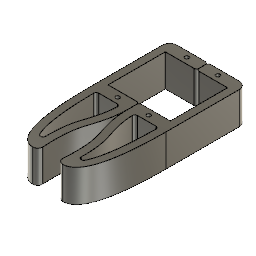
leg2 (Autodesk Fusion 360 design; units mm, degrees)
Autodesk Fusion 360 part; units mm, degrees
sketch "Sketch1" plane through (0, 0, 0) normal (0, 0, 1) x (1, 0, 0)
  line L0 (5.25, 11.5) -> (-6.25, 11.5)
  line L1 (-6.25, 11.5) -> (-6.25, -11.5)
  line L2 (-6.25, -11.5) -> (5.25, -11.5)
  line L3 (-9.25, 13.25) -> (-9.25, -16.25)
  line L4 (6.25, 12.5) -> (6.25, 15.25)
  line L5 (6.25, -12.5) -> (6.25, -16.25)
  line L6 (5.25, 16.25) -> (-6.25, 16.25)
  circle A0 centre (0, 13.9) radius 0.8
  circle A1 centre (0, -13.9) radius 0.8
  spline S0 degree 5 poles (6.25, -16.25) (6.25, -16.6676) (6.2357, -17.5036) (6.1715, -18.7605) (6.0031, -20.434) (5.6739, -22.4784) (5.2523, -24.4268) (4.7694, -26.2419) (4.2577, -27.9159) (3.7493, -29.4897) (3.2734, -31.0346) (2.8556, -32.634) (2.516, -34.367) (2.2668, -36.2872) (2.1131, -38.4227) (2.0561, -40.7853) (2.087, -42.8585) (2.1522, -44.515) (2.2143, -45.6642) (2.25, -46.25) knots 0 0 0 0 0 0 0.066667 0.133333 0.2 0.266667 0.333333 0.4 0.466667 0.533333 0.6 0.666667 0.733333 0.8 0.866667 0.933333 1 1 1 1 1 1
  arc A2 (0.25, -48.25) -> (2.25, -46.25) centre (0.25, -46.25) ccw
  spline S1 degree 5 poles (-9.25, -16.25) (-9.25, -17.2508) (-9.2353, -19.2506) (-9.1693, -22.2447) (-8.9897, -26.2076) (-8.5912, -31.003) (-7.9895, -35.4883) (-7.1545, -39.4912) (-6.0655, -42.8464) (-4.722, -45.4219) (-3.1673, -47.1742) (-1.8215, -47.9565) (-0.7899, -48.2233) (-0.0974, -48.264) (0.25, -48.25) knots 0 0 0 0 0 0 0.1 0.2 0.3 0.4 0.5 0.6 0.7 0.8 0.9 1 1 1 1 1 1
  line L7 (6.25, -13) -> (6.25, -19.5)
  line L8 (-9.25, -12) -> (-9.25, -20.5)
  line L9 (-2.6364, -48.3662) -> (3.1364, -48.1338)
  spline S2 degree 3 poles (-6.2471, -17.2558) (-6.2233, -21.3469) (-6.0529, -25.437) (-5.6953, -29.2432) (-5.3067, -33.3791) (-4.6726, -37.1464) (-3.8118, -39.8822) (-3.4994, -40.8752) (-3.1573, -41.7234) (-2.8107, -42.4245) knots 0.020453 0.020453 0.020453 0.020453 0.27 0.27 0.27 0.541159 0.541159 0.541159 0.639581 0.639581 0.639581 0.639581
  spline S3 degree 3 poles (3.2295, -17.2889) (3.1506, -19.3134) (2.85, -21.3675) (2.4217, -23.2564) (2.0271, -24.9967) (1.5393, -26.5428) (1.0455, -28.106) (0.5017, -29.8277) (-0.0499, -31.6576) (-0.4062, -33.8312) (-0.7884, -36.1626) (-0.9513, -38.8586) (-0.9144, -41.9695) knots 0.036628 0.036628 0.036628 0.036628 0.25 0.25 0.25 0.446598 0.446598 0.446598 0.663121 0.663121 0.663121 0.895358 0.895358 0.895358 0.895358
  line L10 (2.2302, -16.25) -> (-5.2471, -16.25)
  arc A3 (-6.25, 16.25) -> (-9.25, 13.25) centre (-6.25, 13.25) ccw
  arc A4 (6.25, 15.25) -> (5.25, 16.25) centre (5.25, 15.25) ccw
  arc A5 (5.25, 11.5) -> (6.25, 12.5) centre (5.25, 12.5) ccw
  arc A6 (6.25, -12.5) -> (5.25, -11.5) centre (5.25, -12.5) ccw
  arc A7 (-2.8107, -42.4245) -> (-0.9144, -41.9695) centre (-1.9143, -41.9814) ccw
  arc A8 (-5.2471, -16.25) -> (-6.2471, -17.2558) centre (-5.2471, -17.25) ccw
  arc A9 (3.2295, -17.2889) -> (2.2302, -16.25) centre (2.2302, -17.25) ccw
  point P0 (4.75, -26.25)
  point P1 (2.75, -33.25)
  point P2 (-5.25, -44.25)
  constraint midpoint L5.end L7
  constraint coincident L5 L7.start
  constraint midpoint L3.end L8
  constraint coincident L3 L8.start
  constraint midpoint A2.start L9
extrude "Extrude1" add sketch "Sketch1" along normal blind 13 makes body 1
extrude "Extrude3" add sketch "Sketch1" along normal blind 5 contours A0 | A1 bodies 1
mirror "Mirror1" about plane through (6.25, 12.5, 0) normal (1, 0, 0) of bodies 1 makes body 2
named bodies: "leg2", "leg2_mirror"
